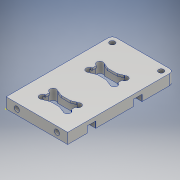
# Autodesk Inventor part: kicker_plate
Saved by Autodesk Inventor 2018 (Build 220112000, 112)
## iProperties
Created: 2019-01-25
Part Number: kicker_plate
Material: Aluminum 6061
Document SubType Name: Modeling
Designer: steve
Density: 2.7 g/cm^3
Appearance: Aluminum - Flat
Author: steve
Autodesk Inventor part; units mm, degrees
ref_plane "YZ Plane" through (0, 0, 0) normal (1, 0, 0) x (0, 1, 0)
ref_plane "XZ Plane" through (0, 0, 0) normal (0, 1, 0) x (-1, 0, 0)
ref_plane "XY Plane" through (0, 0, 0) normal (0, 0, 1) x (1, 0, 0)
sketch "Sketch1" plane through (0, 0, 0) normal (0, 0, 1) x (1, 0, 0)
  line L0 (0, 0) -> (29.1, 0)
  line L1 (29.1, 0) -> (29.1, 44.2)
  line L2 (29.1, 44.2) -> (0, 44.2)
  line L3 (0, 44.2) -> (0, 0)
  dimension "d0" = 29.1
  dimension "d1" = 44.2
  constraints: 8 end point, 2 parallel, 1 horizontal, 1 perpendicular
  measures "d0" distance of L1.end L2.end
  measures "d1" distance of L0.end L1.end
extrude "Extrusion1" add sketch "Sketch1" along normal blind 5
sketch "Sketch2" plane through (0, 0, 5) normal (0, 0, 1) x (1, 0, 0)
  line L0 (29.1, 44.2) -> (0, 44.2) construction
  line L1 (14.55, 44.2) -> (14.55, -5.4706) construction
  line L2 (-11.1615, 33.15) -> (47.7299, 33.15) construction
  line L3 (20.6, 30.6) -> (8.5, 30.6) construction
  line L4 (8.5, 30.6) -> (8.5, 35.7) construction
  line L5 (8.5, 35.7) -> (20.6, 35.7) construction
  line L6 (20.6, 35.7) -> (20.6, 30.6) construction
  line L7 (20.6, 30.6) -> (8.5, 35.7) construction
  line L8 (8.5, 30.6) -> (20.6, 35.7) construction
  line L9 (7.6, 29.7) -> (9.8127, 29.7) construction
  line L10 (21.6, 29.7) -> (21.6, 31.6109) construction
  line L11 (21.6, 36.7) -> (19.3787, 36.7) construction
  line L12 (7.6, 36.7) -> (7.6, 34.5787) construction
  line L13 (7.6, 36.7) -> (13.2917, 31.0083) construction
  arc A0 (8.5, 34.148) -> (9.7213, 34.5787) centre (8.6607, 35.6393) ccw construction
  line L14 (7.6, 34.5787) -> (8.6607, 35.6393) construction
  line L15 (8.6607, 35.6393) -> (9.7213, 36.7) construction
  arc A1 (18.9406, 35.7) -> (19.0596, 35.0508) centre (20.4393, 35.6393) ccw construction
  arc A2 (10.1594, 30.6) -> (10.0404, 31.2492) centre (8.6607, 30.6607) ccw construction
  arc A3 (20.6, 32.152) -> (19.0596, 31.2492) centre (20.4393, 30.6607) ccw construction
  line L16 (7.6, 34.5787) -> (7.6, 31.7213)
  line L17 (9.7213, 36.7) -> (7.6, 36.7) construction
  line L18 (7.6, 31.7213) -> (7.6, 29.7) construction
  line L19 (9.8127, 29.7) -> (19.2873, 29.7)
  line L20 (19.2873, 29.7) -> (21.6, 29.7) construction
  line L21 (21.6, 31.6109) -> (21.6, 34.6891)
  line L22 (21.6, 34.6891) -> (21.6, 36.7) construction
  line L23 (19.3787, 36.7) -> (9.7213, 36.7)
  arc A4 (7.6, 34.5787) -> (8.5, 34.148) centre (8.6607, 35.6393) ccw construction
  arc A5 (9.7213, 34.5787) -> (10.0404, 35.0508) centre (8.6607, 35.6393) ccw construction
  arc A6 (10.0404, 35.0508) -> (10.1594, 35.7) centre (8.6607, 35.6393) ccw construction
  arc A7 (10.1594, 35.7) -> (9.7213, 36.7) centre (8.6607, 35.6393) ccw construction
  arc A8 (9.7213, 36.7) -> (7.6, 34.5787) centre (8.6607, 35.6393) ccw
  arc A9 (19.3787, 36.7) -> (18.9406, 35.7) centre (20.4393, 35.6393) ccw construction
  arc A10 (19.0596, 35.0508) -> (20.6, 34.148) centre (20.4393, 35.6393) ccw construction
  arc A11 (20.6, 34.148) -> (21.6, 34.6891) centre (20.4393, 35.6393) ccw construction
  arc A12 (21.6, 34.6891) -> (19.3787, 36.7) centre (20.4393, 35.6393) ccw
  arc A13 (21.6, 31.6109) -> (20.6, 32.152) centre (20.4393, 30.6607) ccw construction
  arc A14 (19.0596, 31.2492) -> (18.9406, 30.6) centre (20.4393, 30.6607) ccw construction
  arc A15 (18.9406, 30.6) -> (19.2873, 29.7) centre (20.4393, 30.6607) ccw construction
  arc A16 (19.2873, 29.7) -> (21.6, 31.6109) centre (20.4393, 30.6607) ccw
  arc A17 (9.8127, 29.7) -> (10.1594, 30.6) centre (8.6607, 30.6607) ccw construction
  arc A18 (10.0404, 31.2492) -> (8.5, 32.152) centre (8.6607, 30.6607) ccw construction
  arc A19 (8.5, 32.152) -> (7.6, 31.7213) centre (8.6607, 30.6607) ccw construction
  arc A20 (7.6, 31.7213) -> (9.8127, 29.7) centre (8.6607, 30.6607) ccw
  line L24 (0, 44.2) -> (0, 0) construction
  line L25 (0, 22.1) -> (51.9869, 22.1) construction
  line L26 (7.6, 9.6213) -> (7.6, 12.4787)
  line L27 (9.8127, 14.5) -> (19.2873, 14.5)
  line L28 (21.6, 12.5891) -> (21.6, 9.5109)
  line L29 (19.3787, 7.5) -> (9.7213, 7.5)
  arc A21 (7.6, 9.6213) -> (9.7213, 7.5) centre (8.6607, 8.5607) ccw
  arc A22 (19.3787, 7.5) -> (21.6, 9.5109) centre (20.4393, 8.5607) ccw
  arc A23 (21.6, 12.5891) -> (19.2873, 14.5) centre (20.4393, 13.5393) ccw
  arc A24 (9.8127, 14.5) -> (7.6, 12.4787) centre (8.6607, 13.5393) ccw
  point P0 (14.55, 33.15)
  dimension "d7" = 8.5
  dimension "d8" = 1
  dimension "d10" = 45
  dimension "d11" = 3
  dimension "d12" = 7
  dimension "d13" = 14
  dimension "d14" = 7.05
  dimension "d15" = 11.05
  constraints: 64 point on circle, 56 end point, 25 centre point, 20 parallel, 17 point on line, 15 symmetric about line, 10 perpendicular, 4 midpoint, 3 horizontal, 1 vertical, 7 other
  measures "d7" distance between parallel lines of L5 L0
  measures "d8" distance between parallel lines of L11 L5
  measures "d10" angle of L11 L13
  measures "d11" diameter of A0
  measures "d12" distance between parallel lines of L19 L23
  measures "d13" distance between parallel lines of L16 L21
  measures "d14" distance from line of point (14.55, 33.15) L21
  measures "d15" distance between parallel lines of L0 L2
extrude "Extrusion2" cut sketch "Sketch2" against normal blind 6
sketch "Sketch3" plane through (0, 44.2, 0) normal (0, 1, 0) x (1, 0, 0)
  line L0 (29.1, 0) -> (0, 0) projected
  line L1 (0, 0) -> (0, -5) projected
  line L2 (29.1, -5) -> (0, -5) projected
  line L3 (29.1, 0) -> (29.1, -5) projected
  point P0 (0, 0)
extrude "Extrusion3" add sketch "Sketch3" along normal blind 6
sketch "Sketch4" plane through (0, 0, 5) normal (0, 0, 1) x (1, 0, 0)
  line L0 (-2.5701, 47.2) -> (43.8381, 47.2) construction
  line L1 (0, 50.2) -> (29.1, 50.2) construction
  line L2 (14.55, 50.2) -> (14.55, 32.7868) construction
  line L3 (3, 50.2) -> (3, 37.5598) construction
  line L4 (0, 0) -> (0, 50.2) construction
  point P0 (3, 47.2)
  point P1 (26.1, 47.2)
  dimension "d20" = 3
  dimension "d21" = 3
  constraints: 6 end point, 3 point on line, 2 vertical, 1 horizontal, 1 midpoint, 1 symmetric about line
  measures "d20" distance between parallel lines of L0 L1
  measures "d21" distance between parallel lines of L4 L3
hole "Hole1" at (3, 47.2, 5) at (26.1, 47.2, 5) direction (0, 0, -1) diameter 2.5 end through all
sketch "Sketch5" plane through (0, 0, 0) normal (0, -1, 0) x (1, 0, 0)
  line L0 (29.1, 0) -> (29.1, 5) construction
  line L1 (23.825, 21.8826) -> (23.825, -12.5528) construction
  line L2 (9.8127, 5) -> (19.2873, 5) construction
  line L3 (14.55, 5) -> (14.55, -18.3203) construction
  line L4 (29.1, 2) -> (-6.5259, 2) construction
  line L5 (29.1, 2.5) -> (-3.9615, 2.5) construction
  point P0 (0, 0)
  point P1 (23.825, 2)
  point P2 (5.275, 2)
  dimension "d29" = 9.275
  dimension "d37" = 0.5
  constraints: 8 end point, 3 point on line, 2 midpoint, 2 vertical, 1 horizontal, 1 parallel, 1 symmetric about line
  measures "d29" distance between parallel lines of L1 L3
  measures "d37" distance between parallel lines of L4 L5
hole "Hole2" [suppressed]
sketch "Sketch6" plane through (0, 0, 5) normal (0, 0, -1) x (-1, 0, 0)
  circle A0 centre (-3, 47.2) radius 1.25 construction
  circle A1 centre (-26.1, 47.2) radius 1.25 construction
  arc A2 (-9.8127, 29.7) -> (-7.6, 31.7213) centre (-8.6607, 30.6607) ccw construction
  line L0 (-9.8127, 29.7) -> (-19.2873, 29.7) construction
  arc A3 (-21.6, 31.6109) -> (-19.2873, 29.7) centre (-20.4393, 30.6607) ccw construction
  line L1 (-21.6, 31.6109) -> (-21.6, 34.6891) construction
  arc A4 (-19.3787, 36.7) -> (-21.6, 34.6891) centre (-20.4393, 35.6393) ccw construction
  line L2 (-19.3787, 36.7) -> (-9.7213, 36.7) construction
  arc A5 (-7.6, 34.5787) -> (-9.7213, 36.7) centre (-8.6607, 35.6393) ccw construction
  line L3 (-7.6, 34.5787) -> (-7.6, 31.7213) construction
  arc A6 (-7.6, 12.4787) -> (-9.8127, 14.5) centre (-8.6607, 13.5393) ccw construction
  line L4 (-7.6, 12.4787) -> (-7.6, 9.6213) construction
  arc A7 (-9.7213, 7.5) -> (-7.6, 9.6213) centre (-8.6607, 8.5607) ccw construction
  line L5 (-9.7213, 7.5) -> (-19.3787, 7.5) construction
  arc A8 (-21.6, 9.5109) -> (-19.3787, 7.5) centre (-20.4393, 8.5607) ccw construction
  line L6 (-21.6, 9.5109) -> (-21.6, 12.5891) construction
  arc A9 (-19.2873, 14.5) -> (-21.6, 12.5891) centre (-20.4393, 13.5393) ccw construction
  line L7 (-19.2873, 14.5) -> (-9.8127, 14.5) construction
  line L8 (0, 0) -> (-29.1, 0) construction
  line L9 (0, 0) -> (0, 50.2) construction
  line L10 (-29.1, 50.2) -> (0, 50.2) construction
  line L11 (-29.1, 0) -> (-29.1, 50.2) construction
  line L12 (-14.55, 14.5) -> (-14.55, 29.7) construction
  line L13 (-14.55, 22.1) -> (-55.4317, 22.1) construction
  line L14 (-19.3787, 7.5) -> (-9.7213, 7.5) construction
  line L15 (-14.55, 7.5) -> (-14.55, 14.5) construction
  line L16 (-21.6, 12.5891) -> (-21.6, 9.5109) construction
  line L17 (-21.6, 11.05) -> (-7.6, 11.05) construction
  line L18 (-20.65, 13.6) -> (-8.55, 13.6) construction
  line L19 (-8.55, 13.6) -> (-8.55, 8.5) construction
  line L20 (-8.55, 8.5) -> (-20.65, 8.5) construction
  line L21 (-20.65, 8.5) -> (-20.65, 13.6) construction
  line L22 (-20.65, 13.6) -> (-8.55, 8.5) construction
  line L23 (-8.55, 13.6) -> (-20.65, 8.5) construction
  circle A10 centre (-8.6607, 8.5607) radius 1.5 construction
  circle A11 centre (-8.6607, 13.5393) radius 1.5 construction
  circle A12 centre (-20.4393, 13.5393) radius 1.5 construction
  arc A13 (-19.2873, 14.5) -> (-21.6, 12.5891) centre (-20.4393, 13.5393) ccw construction
  circle A14 centre (-20.4393, 8.5607) radius 1.5 construction
  line L24 (-8.0767, 9.9423) -> (-19.8553, 14.921) construction
  line L25 (-9.2447, 14.921) -> (-21.0233, 9.9423) construction
  line L26 (-9.2447, 7.179) -> (-21.0233, 12.1577) construction
  line L27 (-19.8553, 7.179) -> (-8.0767, 12.1577) construction
  line L28 (-8.55, 10.1424) -> (-8.55, 11.9576)
  line L29 (-12.3699, 13.6) -> (-16.7301, 13.6)
  line L30 (-20.65, 11.9999) -> (-20.65, 10.1001)
  line L31 (-16.7301, 8.5) -> (-12.3699, 8.5)
  line L32 (-8.55, 11.9576) -> (-8.0767, 12.1577)
  line L33 (-8.55, 10.1424) -> (-8.0767, 9.9423)
  line L34 (-12.3699, 8.5) -> (-10.0041, 7.5)
  line L35 (-16.7301, 8.5) -> (-19.0959, 7.5)
  line L36 (-20.65, 10.1001) -> (-21.0233, 9.9423)
  line L37 (-20.65, 11.9999) -> (-21.0233, 12.1577)
  line L38 (-16.7301, 13.6) -> (-18.8594, 14.5)
  line L39 (-12.3699, 13.6) -> (-10.2406, 14.5)
  line L40 (-9.8127, 14.5) -> (-19.2873, 14.5) projected
  line L41 (-10.0041, 7.5) -> (-19.0959, 7.5)
  line L42 (-10.2406, 14.5) -> (-18.8594, 14.5)
  arc A15 (-8.0767, 12.1577) -> (-7.6, 12.4787) centre (-8.6607, 13.5393) ccw
  arc A16 (-7.6, 9.6213) -> (-8.0767, 9.9423) centre (-8.6607, 8.5607) ccw
  arc A17 (-21.0233, 9.9423) -> (-21.6, 9.5109) centre (-20.4393, 8.5607) ccw
  arc A18 (-21.6, 12.5891) -> (-21.0233, 12.1577) centre (-20.4393, 13.5393) ccw
  line L43 (-7.6, 9.6213) -> (-7.6, 12.4787) projected
  line L44 (-7.6, 9.6213) -> (-7.6, 12.4787)
  line L45 (-21.6, 12.5891) -> (-21.6, 9.5109)
  line L46 (-8.55, 34.0576) -> (-8.55, 32.2424)
  line L47 (-12.3699, 30.6) -> (-16.7301, 30.6)
  line L48 (-20.65, 32.2001) -> (-20.65, 34.0999)
  line L49 (-16.7301, 35.7) -> (-12.3699, 35.7)
  line L50 (-8.55, 32.2424) -> (-8.0767, 32.0423)
  line L51 (-8.55, 34.0576) -> (-8.0767, 34.2577)
  line L52 (-12.3699, 35.7) -> (-10.0041, 36.7)
  line L53 (-16.7301, 35.7) -> (-19.0959, 36.7)
  line L54 (-20.65, 34.0999) -> (-21.0233, 34.2577)
  line L55 (-20.65, 32.2001) -> (-21.0233, 32.0423)
  line L56 (-16.7301, 30.6) -> (-18.8594, 29.7)
  line L57 (-12.3699, 30.6) -> (-10.2406, 29.7)
  line L58 (-10.0041, 36.7) -> (-19.0959, 36.7)
  line L59 (-10.2406, 29.7) -> (-18.8594, 29.7)
  arc A19 (-7.6, 31.7213) -> (-8.0767, 32.0423) centre (-8.6607, 30.6607) ccw
  arc A20 (-8.0767, 34.2577) -> (-7.6, 34.5787) centre (-8.6607, 35.6393) ccw
  arc A21 (-21.6, 34.6891) -> (-21.0233, 34.2577) centre (-20.4393, 35.6393) ccw
  arc A22 (-21.0233, 32.0423) -> (-21.6, 31.6109) centre (-20.4393, 30.6607) ccw
  line L60 (-7.6, 34.5787) -> (-7.6, 31.7213)
  line L61 (-21.6, 31.6109) -> (-21.6, 34.6891)
  point P0 (-14.6, 11.05)
  dimension "d38" = 5.1
  dimension "d39" = 12.1
  constraints: 92 end point, 25 point on line, 24 point on circle, 21 symmetric about line, 12 centre point, 11 tangent, 9 midpoint, 8 coincident, 3 collinear, 3 horizontal, 2 concentric, 2 parallel, 2 perpendicular, 4 other
  measures "d38" distance between parallel lines of L18 L20
  measures "d39" distance between parallel lines of L19 L21
extrude "Extrusion4" add sketch "Sketch6" along normal blind 1
fillet "Fillet1" radius 2 2 edges at (29.1, 50.2, 2.5) (0, 50.2, 2.5)
sketch "Sketch7" plane through (0, 0, 0) normal (0, 0, -1) x (-1, 0, 0)
  line L0 (-36.6097, 22.2) -> (17.6327, 22.2) construction
  line L1 (-9.8127, 29.7) -> (-19.2873, 29.7) construction
  line L2 (-19.2873, 14.5) -> (-9.8127, 14.5) construction
  line L3 (-21.6, 31.6109) -> (-21.6, 34.6891) construction
  line L4 (-21.6, 33.15) -> (3.7466, 33.15) construction
  line L5 (-6.6, 42.634) -> (-6.6, 22.2) construction
  line L6 (-7.6, 34.5787) -> (-7.6, 31.7213) construction
  circle A0 centre (-5.1, 33.15) radius 1.5 construction
  line L7 (-26.1, 40.379) -> (-26.1, 24.0033) construction
  line L8 (-21.6, 33.15) -> (-32.2264, 33.15) construction
  line L9 (-29.1, 0) -> (-29.1, 48.2) construction
  line L10 (-26.1, 31.65) -> (-29.1, 31.65) construction
  line L11 (-29.1, 31.65) -> (-29.1, 34.65) construction
  line L12 (-29.1, 34.65) -> (-26.1, 34.65) construction
  line L13 (-26.1, 34.65) -> (-26.1, 31.65) construction
  line L14 (-26.1, 31.65) -> (-29.1, 34.65) construction
  line L15 (-29.1, 31.65) -> (-26.1, 34.65) construction
  arc A1 (-27.6, 31.65) -> (-27.6, 34.65) centre (-27.6, 33.15) ccw construction
  line L16 (-27.6, 34.65) -> (-29.1, 34.65) construction
  line L17 (-29.1, 34.65) -> (-29.1, 31.65) construction
  line L18 (-29.1, 31.65) -> (-27.6, 31.65) construction
  line L19 (-21.6, 11.25) -> (3.7466, 11.25) construction
  line L20 (-6.6, 1.766) -> (-6.6, 22.2) construction
  circle A2 centre (-5.1, 11.25) radius 1.5 construction
  line L21 (-26.1, 12.75) -> (-29.1, 12.75) construction
  line L22 (-29.1, 12.75) -> (-29.1, 9.75) construction
  line L23 (-29.1, 9.75) -> (-26.1, 9.75) construction
  line L24 (-26.1, 9.75) -> (-26.1, 12.75) construction
  line L25 (-26.1, 12.75) -> (-29.1, 9.75) construction
  line L26 (-29.1, 12.75) -> (-26.1, 9.75) construction
  arc A3 (-27.6, 9.75) -> (-27.6, 12.75) centre (-27.6, 11.25) ccw construction
  line L27 (-27.6, 9.75) -> (-29.1, 9.75) construction
  line L28 (-29.1, 9.75) -> (-29.1, 12.75) construction
  line L29 (-29.1, 12.75) -> (-27.6, 12.75) construction
  line L30 (-4.6, 11.25) -> (-0.0677, 11.25) construction
  line L31 (-4.6, 9.25) -> (-0.0677, 9.25)
  line L32 (-0.0677, 13.25) -> (-4.6, 13.25)
  arc A4 (-4.6, 13.25) -> (-4.6, 9.25) centre (-4.6, 11.25) ccw
  arc A5 (-0.0677, 9.25) -> (-0.0677, 13.25) centre (-0.0677, 11.25) ccw
  line L33 (0, 0) -> (-29.1, 0) construction
  line L34 (-14.55, 0) -> (-14.55, 76.2221) construction
  line L35 (-24.5, 9.25) -> (-29.0323, 9.25)
  line L36 (-29.0323, 13.25) -> (-24.5, 13.25)
  arc A6 (-24.5, 9.25) -> (-24.5, 13.25) centre (-24.5, 11.25) ccw
  arc A7 (-29.0323, 13.25) -> (-29.0323, 9.25) centre (-29.0323, 11.25) ccw
  line L37 (-4.6, 35.15) -> (-0.0677, 35.15)
  line L38 (-0.0677, 31.15) -> (-4.6, 31.15)
  arc A8 (-4.6, 35.15) -> (-4.6, 31.15) centre (-4.6, 33.15) ccw
  arc A9 (-0.0677, 31.15) -> (-0.0677, 35.15) centre (-0.0677, 33.15) ccw
  arc A10 (-29.0323, 35.15) -> (-29.0323, 31.15) centre (-29.0323, 33.15) ccw
  line L39 (-29.0323, 31.15) -> (-24.5, 31.15)
  arc A11 (-24.5, 31.15) -> (-24.5, 35.15) centre (-24.5, 33.15) ccw
  line L40 (-24.5, 35.15) -> (-29.0323, 35.15)
  point P0 (-2.3338, 11.25)
  dimension "d43" = 7.5
  dimension "d44" = 15.2
  dimension "d45" = 1
  dimension "d46" = 3
  dimension "d47" = 4.5
  dimension "d48" = 3
  dimension "d61" = 4
  constraints: 72 end point, 30 symmetric about line, 20 point on circle, 12 centre point, 9 midpoint, 7 point on line, 6 tangent, 4 collinear, 4 horizontal, 3 parallel, 3 vertical, 2 coincident, 1 perpendicular, 8 other
  measures "d43" distance between parallel lines of L0 L1
  measures "d44" distance between parallel lines of L2 L1
  measures "d45" distance between parallel lines of L6 L5
  measures "d46" diameter of A0
  measures "d47" distance between parallel lines of L7 L3
  measures "d48" distance between parallel lines of L10 L12
  measures "d61" distance between parallel lines of L32 L31
sketch "Sketch8" plane through (0, 0, 0) normal (0, -1, 0) x (1, 0, 0)
  line L0 (0, 0) -> (0, 5) construction
  line L1 (0, 2.5) -> (29.1, 2.5) construction
  line L2 (29.1, 0) -> (29.1, 5) construction
  line L3 (9.8127, 0) -> (19.2873, 0) construction
  line L4 (14.55, 0) -> (14.55, 13.5934) construction
  point P0 (24.05, 2.5)
  point P1 (5.05, 2.5)
  dimension "d53" = 9.5
  constraints: 4 end point, 3 midpoint, 1 point on line, 1 symmetric about line, 1 vertical
  measures "d53" distance from line of L4 point (24.05, 2.5)
hole "Hole3" at (24.05, 0, 2.5) at (5.05, 0, 2.5) direction (0, 1, 0) diameter 2.459 depth 8.8 tip angle 118 thread size "M3x0.5" class "6H" standard "ISO Metric profile"
sketch "Sketch9" plane through (0, 0, 0) normal (0, 0, -1) x (-1, 0, 0)
  point P0 (0, 0)
extrude "Extrusion7" cut sketch "Sketch7" against normal blind 3
body "Solid1"
